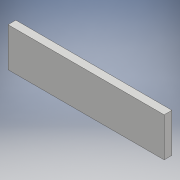
# Autodesk Inventor part: BedBoard
Saved by Autodesk Inventor 2017 (Build 210142000, 142)
## iProperties
Created: 2019-07-06
Part Number: BedBoard
Material: Generic
Document SubType Name: Modeling
Designer: Ole Simmering
Density: 1 g/cm^3
Appearance: Default
Author: Ole Simmering
Autodesk Inventor part; units mm, degrees
ref_plane "YZ Plane" through (0, 0, 0) normal (1, 0, 0) x (0, 1, 0)
sketch "Sketch1" plane through (0, 0, 0) normal (1, 0, 0) x (0, 1, 0)
  line L0 (0, 0) -> (25.4, 0)
  line L1 (25.4, 0) -> (25.4, 127)
  line L2 (25.4, 127) -> (0, 127)
  line L3 (0, 127) -> (0, 0)
  dimension "d2" = 127
  dimension "d3" = 25.4
  constraints: 8 end point, 2 parallel, 1 horizontal, 1 perpendicular
  measures "d2" distance between parallel lines of L0 L2
  measures "d3" distance between parallel lines of L3 L1
extrude "Extrusion1" add sketch "Sketch1" along normal blind 508
ref_plane "Work Plane1" through (0, 0, 63.5) normal (0, 0, 1) x (1, 0, 0)
ref_plane "Work Plane2" through (254, 0, 0) normal (-1, 0, 0) x (0, 0, 1)
body "Solid1"
